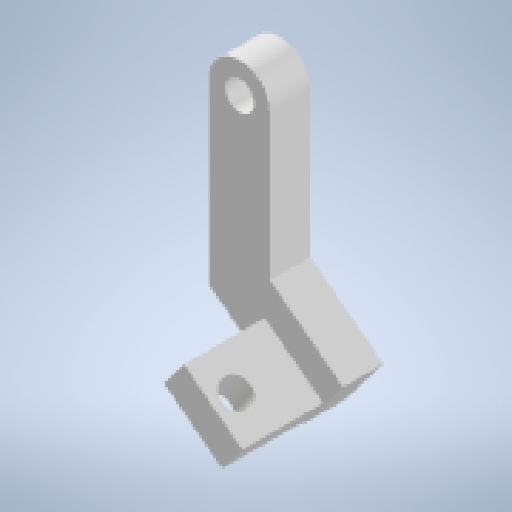
# Autodesk Inventor part: mirror_arm_2
Saved by Autodesk Inventor 2025.1 (Build 291241020, 241B)
## iProperties
Created: 2024-10-13
Part Number: mirror_arm_2
Material: Ogólny
Document SubType Name: Modeling
Designer: zychlix
Density: 1 g/cm^3
Appearance: Domyślna
Author: zychlix
Autodesk Inventor part; units mm, degrees
ref_plane "YZ Plane" through (0, 0, 0) normal (1, 0, 0) x (0, 1, 0)
ref_plane "XZ Plane" through (0, 0, 0) normal (0, 1, 0) x (-1, 0, 0)
ref_plane "XY Plane" through (0, 0, 0) normal (0, 0, 1) x (1, 0, 0)
sketch "Szkic1" plane through (0, 0, 0) normal (0, 0, 1) x (1, 0, 0)
  circle A0 centre (26.2, 0.975) radius 1.45 projected
  circle A1 centre (26.2, 0.975) radius 3
  line L0 (29.2, 0.975) -> (29.2, -8.7925)
  line L1 (23.2, -7.0757) -> (23.2, 0.975)
  line L2 (16.8275, -11.925) -> (-16.8275, 13.875) construction
  line L3 (23.2, -7.0757) -> (23.2, -16.8102)
  line L4 (23.2, -16.8102) -> (32.5797, -24.0007)
  line L5 (32.5797, -24.0007) -> (36.4465, -18.9567)
  line L6 (36.4465, -18.9567) -> (29.2, -13.4015)
  line L7 (29.2, -13.4015) -> (29.2, -8.7925)
  point P0 (0, 0)
  point P1 (29.2, -14.7925)
  point P2 (18.5681, -14.7925)
  point P3 (15.1107, -9.0757)
  point P4 (23.2, -9.0757)
  dimension "d5" = 6
  dimension "d12" = 2
  dimension "d13" = 6
  constraints: 14 end point, 2 perpendicular, 2 point on circle, 2 point on line, 2 tangent, 2 vertical, 1 centre point, 1 coincident, 1 collinear
  measures "d5" distance of L0.end point (29.2, -14.793)
  measures "d12" distance of L1.start point (23.2, -9.076)
  measures "d13" diameter of A1
extrude "Wyciągnięcie proste1" add sketch "Szkic1" along normal blind 4
sketch "Szkic4" plane through (0, 0, 4) normal (0, 0, 1) x (1, 0, 0)
  line L0 (34.4685, -21.3117) -> (28.6942, -16.8851)
  line L1 (16.8275, -11.925) -> (-16.8275, 13.875) construction
  line L2 (28.6942, -16.8851) -> (26.6967, -19.4907)
  line L3 (26.6967, -19.4907) -> (32.471, -23.9174)
  line L4 (32.471, -23.9174) -> (34.4685, -21.3117)
  line L5 (15.6301, -11.0071) -> (20.5681, -14.7925) projected
  line L6 (17.1107, -9.0757) -> (15.6301, -11.0071) projected
  point P0 (0, 0)
  constraints: 8 end point, 1 collinear, 1 parallel, 1 perpendicular
extrude "Wyciągnięcie proste2" add sketch "Szkic4" along normal blind 8 and the other way blind 4
sketch "Szkic6" plane through (23.2, -16.8102, 0) normal (-0.6084, -0.7936, 0) x (0.7936, -0.6084, 0)
  circle A0 centre (8.0439, 9.69) radius 1.45
  point P0 (-28.6395, 0)
  dimension "d21" = 2.9
  constraints: 1 centre point
  measures "d21" diameter of A0
extrude "Wyciągnięcie proste4" cut sketch "Szkic6" against normal blind 7
equation "\"d12\" = d11"
equation "\"d11\" = d7"
equation "\"d7\" = 2"
